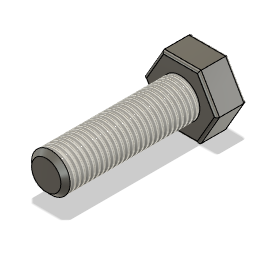
0.160.4837 - Boulon H - M16-55_38 (Autodesk Fusion 360 design; units mm, degrees)
Autodesk Fusion 360 part; units mm, degrees
sketch "Sketch1" plane through (0, 0, 0) normal (0, 0, 1) x (1, 0, 0)
  circle A0 centre (0, 0) radius 8
  line L0 (0, 0) -> (0, 8) construction
  line L1 (0, 0) -> (-8, 0) construction
  line L2 (0, 0) -> (8, 0) construction
  line L3 (0, 0) -> (0, -8) construction
  line L4 (-4.6188, 8) -> (-9.2376, 0) construction
  line L5 (-9.2376, 0) -> (-4.6188, -8) construction
  line L6 (-4.6188, -8) -> (4.6188, -8) construction
  line L7 (4.6188, -8) -> (9.2376, 0) construction
  line L8 (9.2376, 0) -> (4.6188, 8) construction
  line L9 (4.6188, 8) -> (-4.6188, 8) construction
  line L10 (-7.5056, -13) -> (7.5056, -13)
  line L11 (7.5056, -13) -> (15.0111, 0)
  line L12 (15.0111, 0) -> (7.5056, 13)
  line L13 (7.5056, 13) -> (-7.5056, 13)
  line L14 (-7.5056, 13) -> (-15.0111, 0)
  line L15 (-15.0111, 0) -> (-7.5056, -13)
  dimension "d1" = 16
  dimension "d4" = 5
  constraint coincident A0.centre L0.start
  constraint coincident A0 L0.end
  constraint vertical L0
  constraint coincident A0 L1.end
  constraint perpendicular L0 L1
  constraint coincident A0 L2.end
  constraint perpendicular L0 L2
  constraint coincident A0 L3.end
  constraint perpendicular L1 L3
  measures "d1" diameter of A0
extrude "Extrude1" add sketch "Sketch1" along normal blind 55 contours A0 makes body 1
extrude "Extrude2" add sketch "Sketch1" against normal blind 12 separate body contours A0 | L10 L11 L12 L13 L14 L15 makes body 2
chamfer "Chamfer1" distance 2 angle 45 1 edges at (-7.4586, -2.8929, 55) on bodies 1
fillet "Fillet1" radius 1 12 edges at (0, 13, 0) (11.2583, 6.5, 0) (0, 13, -12) (11.2583, 6.5, -12) (11.2583, -6.5, 0) (11.2583, -6.5, -12) (0, -13, 0) (0, -13, -12) (-11.2583, -6.5, 0) (-11.2583, -6.5, -12) (-11.2583, 6.5, 0) (-11.2583, 6.5, -12) on bodies 2
thread "Thread1" "ISO Metric profile 16.0 M16x2 6g" major diameter 15.822 minor diameter 13.534 pitch 2 angle 60 resizes the face on face at (7.9901, -0.3988, 35.3333) on bodies 1
